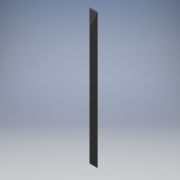
# Autodesk Inventor part: 3 x 3 angle 45 .25 steel-54
Saved by Autodesk Inventor 2019 (Build 230136000, 136)
## iProperties
Created: 2017-12-19
Part Number: 3 x 3 angle 45 .25 steel-54
Material: Steel
Document SubType Name: Modeling
Designer: torba
Density: 7.85 g/cm^3
Appearance: Dark Gray
Author: torba
Autodesk Inventor part; units mm, degrees
ref_plane "YZ Plane" through (0, 0, 0) normal (1, 0, 0) x (0, 1, 0)
ref_plane "XZ Plane" through (0, 0, 0) normal (0, 1, 0) x (-1, 0, 0)
ref_plane "XY Plane" through (0, 0, 0) normal (0, 0, 1) x (1, 0, 0)
sketch "Sketch1" plane through (0, 0, 0) normal (0, 1, 0) x (-1, 0, 0)
  line L0 (0, 0) -> (0, -76.2)
  line L1 (0, -76.2) -> (76.2, -76.2)
  line L2 (76.2, -76.2) -> (76.2, -69.85)
  line L3 (76.2, -69.85) -> (6.35, -69.85)
  line L4 (6.35, -69.85) -> (6.35, 0)
  line L5 (6.35, 0) -> (0, 0)
  dimension "d0" = 76.2
  dimension "d1" = 76.2
  dimension "d2" = 6.35
  dimension "d3" = 6.35
  constraints: 12 end point, 5 perpendicular, 1 vertical
  measures "d0" distance of L0.start L0.end
  measures "d1" distance of L0.end L1.end
  measures "d2" distance between parallel lines of L1 L3
  measures "d3" distance between parallel lines of L0 L4
extrude "Extrusion1" add sketch "Sketch1" along normal blind 1371.6
sketch "Sketch3" plane through (0, 0, 0) normal (1, 0, 0) x (0, 0, -1)
  line L0 (0, 0) -> (76.2, 0) projected
  line L1 (76.2, 0) -> (76.2, 1371.6) projected
  line L2 (0, 1371.6) -> (76.2, 1371.6) projected
  line L3 (0, 0) -> (0, 1371.6) projected
  line L4 (0, 0) -> (76.2, 0)
  line L5 (76.2, 0) -> (76.2, 76.2)
  line L6 (76.2, 76.2) -> (0, 76.2)
  line L7 (0, 76.2) -> (0, 0)
  line L8 (0, 1371.6) -> (76.2, 1371.6)
  line L9 (76.2, 1371.6) -> (76.2, 1295.4)
  line L10 (76.2, 1295.4) -> (0, 1295.4)
  line L11 (0, 1295.4) -> (0, 1371.6)
  line L12 (0, 1295.4) -> (76.2, 1371.6)
  line L13 (0, 76.2) -> (76.2, 0)
  dimension "d22" = 76.2
  dimension "d23" = 76.2
  dimension "d24" = 76.2
  dimension "d25" = 76.2
  constraints: 20 end point, 4 parallel, 2 horizontal, 2 perpendicular
  measures "d22" distance of L6.end L5.end
  measures "d23" distance of L5.end L4.end
  measures "d24" distance of L9.end L10.end
  measures "d25" distance of L8.end L9.end
extrude "Extrusion3" cut sketch "Sketch3" against normal up to next contours L3 L13 L0 | L3 L2 L12
fillet "Fillet1" radius 3.175 2 edges at (-6.35, 685.8, 0) (-76.2, 685.8, -69.85)
body "Solid1"
